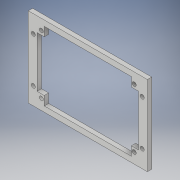
# Autodesk Inventor part: Part14
Saved by Autodesk Inventor 2019 (Build 230136000, 136)
## iProperties
Created: 2019-12-12
Part Number: Part14
Material: Generic
Document SubType Name: Modeling
Designer: dacastro
Density: 1 g/cm^3
Appearance: Default
Author: dacastro
Autodesk Inventor part; units mm, degrees
ref_plane "YZ Plane" through (0, 0, 0) normal (1, 0, 0) x (0, 1, 0)
ref_plane "XZ Plane" through (0, 0, 0) normal (0, 1, 0) x (-1, 0, 0)
ref_plane "XY Plane" through (0, 0, 0) normal (0, 0, 1) x (1, 0, 0)
sketch "Sketch1" plane through (0, 0, 0) normal (0, 0, 1) x (1, 0, 0)
  line L0 (-41, -27.5) -> (41, -27.5)
  line L1 (41, -27.5) -> (41, 27.5)
  line L2 (41, 27.5) -> (-41, 27.5)
  line L3 (-41, 27.5) -> (-41, -27.5)
  line L4 (-41, -27.5) -> (41, 27.5) construction
  line L5 (41, -27.5) -> (-41, 27.5) construction
  line L6 (-37.5, -15.5) -> (37.5, -15.5) construction
  line L7 (37.5, -15.5) -> (37.5, 15.5) construction
  line L8 (37.5, 15.5) -> (-37.5, 15.5) construction
  line L9 (-37.5, 15.5) -> (-37.5, -15.5) construction
  line L10 (-37.5, -15.5) -> (37.5, 15.5) construction
  line L11 (37.5, -15.5) -> (-37.5, 15.5) construction
  line L12 (-32, -20.25) -> (32, -20.25) construction
  line L13 (32, -20.25) -> (32, 20.25) construction
  line L14 (32, 20.25) -> (-32, 20.25) construction
  line L15 (-32, 20.25) -> (-32, -20.25) construction
  line L16 (-32, -20.25) -> (32, 20.25) construction
  line L17 (32, -20.25) -> (-32, 20.25) construction
  line L18 (0, -23.75) -> (30, -23.75)
  line L19 (30, -23.75) -> (30, -17.5)
  line L20 (30, -17.5) -> (35, -17.5)
  line L21 (35, -17.5) -> (35, 0)
  line L22 (0, 0) -> (0, -23.75) construction
  line L23 (0, 0) -> (35, 0) construction
  line L24 (0, -23.75) -> (-30, -23.75)
  line L25 (-30, -23.75) -> (-30, -17.5)
  line L26 (-30, -17.5) -> (-35, -17.5)
  line L27 (-35, -17.5) -> (-35, 0)
  line L28 (0, 23.75) -> (30, 23.75)
  line L29 (30, 23.75) -> (30, 17.5)
  line L30 (30, 17.5) -> (35, 17.5)
  line L31 (35, 17.5) -> (35, 0)
  line L32 (0, 23.75) -> (-30, 23.75)
  line L33 (-30, 23.75) -> (-30, 17.5)
  line L34 (-30, 17.5) -> (-35, 17.5)
  line L35 (-35, 17.5) -> (-35, 0)
  dimension "d0" = 55
  dimension "d1" = 82
  dimension "d2" = 31
  dimension "d3" = 75
  dimension "d4" = 64
  dimension "d5" = 40.5
  dimension "d7" = 60
  dimension "d8" = 70
  dimension "d9" = 47.5
  dimension "d10" = 35
  constraints: 72 end point, 11 symmetric about line, 8 coincident, 7 perpendicular, 6 midpoint, 6 parallel, 4 horizontal, 1 vertical
  measures "d0" distance of L0.end L1.end
  measures "d1" distance of L1.end L2.end
  measures "d2" distance of L6.end L7.end
  measures "d3" distance of L7.end L8.end
  measures "d4" distance of L13.end L14.end
  measures "d5" distance of L12.end L13.end
  measures "d7" diameter of L19 L22
  measures "d8" diameter of L21 L22
  measures "d9" diameter of L18 L23
  measures "d10" diameter of L20 L23
extrude "Extrusion1" add sketch "Sketch1" along normal blind 3
hole "Hole1" at (-32, 20.25, 0) at (-37.5, 15.5, 0) at (-37.5, -15.5, 0) at (-32, -20.25, 0) at (32, -20.25, 0) at (37.5, -15.5, 0) at (37.5, 15.5, 0) at (32, 20.25, 0) direction (0, 0, 1) diameter 2.7 end through all
body "Solid1"
